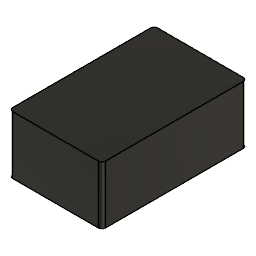
CRTC2025场地（发加工版）V0.1 (Autodesk Fusion 360 archive; units mm, degrees)
design "2*2连接块"
part number: 2025-10-05-20-54-49-775
part number: 2025-10-05-20-58-51-837
part number: 2025-10-05-21-00-41-640
Autodesk Fusion 360 part; units mm, degrees
note: some values were not read from the file. Chosen so that the rebuilt part matches the saved one: which bodies a step acts on.
sketch "草图1" plane through (0, 0, 0) normal (0, 0, 1) x (1, 0, 0)
  line L0 (-16, 25) -> (16, 25)
  line L1 (16, 25) -> (16, -25)
  line L2 (16, -25) -> (-16, -25)
  line L3 (-16, -25) -> (-16, 25)
  line L4 (-16, 25) -> (16, -25) construction
  line L5 (16, 25) -> (-16, -25) construction
  dimension "d1" = 50
  dimension "d2" = 32
  constraint horizontal L0
  constraint perpendicular L0 L1
  constraint parallel L0 L2
  constraint parallel L1 L3
  constraint coincident L4 origin
  constraint coincident L5 origin
  measures "d1" distance of L0.end L1.end
  measures "d2" distance of L1.end L2.end
extrude "拉伸1" add sketch "草图1" along normal blind 20 makes body 1
sketch "草图2" plane through (0, 0, 0) normal (0, 0, -1) x (1, 0, 0)
  line L0 (16, 25) -> (-16, 25)
  line L1 (-16, 25) -> (-16, -25)
  line L2 (-16, -25) -> (16, -25)
  line L3 (16, -25) -> (16, 25)
  line L4 (0, 25) -> (0, -25) construction
  line L5 (0, 0) -> (-16, 0) construction
  circle A0 centre (-8, 12.5) radius 4.05
  circle A1 centre (-8, -12.5) radius 4.05
  circle A2 centre (8, 12.5) radius 4.05
  circle A3 centre (8, -12.5) radius 4.05
  dimension "d5" = 25
  dimension "d6" = 8.1
  dimension "d7" = 16
  constraint midpoint L0 L4.start
  constraint midpoint L2 L4.end
  constraint coincident L5.start origin
  constraint midpoint L1 L5.end
  constraint symmetric L5 A0 A1
  constraint symmetric L4 A0 A2
  constraint symmetric L4 A1 A3
  measures "d5" distance of A0.centre A1.centre
  measures "d6" diameter of A0
  measures "d7" distance of A0.centre A2.centre
extrude "拉伸2" cut sketch "草图2" against normal blind 5.2 contours A0 | A1 | A2 | A3 bodies 1
chamfer "倒角1" distance 0.5 angle 45 4 edges at (-11.7759, -13.9645, 0) (4.2241, -13.9645, 0) (4.2241, 11.0355, 0) (-11.7759, 11.0355, 0) measured on face at (-1.9917, -2.9975, 0) measured on face at (-1.9917, -2.9975, 0) measured on face at (-1.9917, -2.9975, 0) measured on face at (-1.9917, -2.9975, 0) on bodies 1
copy_body "实体->零部件1" bodies 1 removing the originals makes body 2 in component "磁吸连接块"
fillet "圆角1" radius 1.2 4 edges at (-16, -25, 10) (-16, 25, 10) (16, 25, 10) (16, -25, 10) on bodies 2 in component "磁吸连接块"
sketch "草图3" plane through (0, 0, 5.2) normal (0, 0, -1) x (1, 0, 0)
  circle A0 centre (-8, -12.5) radius 4.05
  circle A1 centre (-8, -12.5) radius 4
  dimension "d14" = 8
  constraint concentric A0 A1
  measures "d14" diameter of A1
extrude "拉伸1'" add sketch "草图3" along normal blind 5 from surface at 0.2 separate body contours A1 makes body 3 in component "8*5铷磁铁"
chamfer "倒角1'" distance 0.2 angle 45 2 edges at (-11.7293, 13.9465, 0) (-11.7293, 13.9465, 5) measured on face at (-6.2388, 11.5344, 0) measured on face at (-4.005, 12.6994, 1.6667) on bodies 3 in component "8*5铷磁铁"
pattern_linear "00000000-0000-0000-0000-000000000000" [suppressed]
component "磁吸连接块" placed x (1, 0, 0) y (0, 1, 0) z (0, 0, 1) at (0, 0, 0)
component "8*5铷磁铁" placed x (1, 0, 0) y (0, 1, 0) z (0, 0, 1) at (0, 0, 0)
component "8*5铷磁铁" placed x (1, 0, 0) y (0, 1, 0) z (0, 0, 1) at (16, 0, 0)
component "8*5铷磁铁" placed x (1, 0, 0) y (0, 1, 0) z (0, 0, 1) at (0, -25, 0)
component "8*5铷磁铁" placed x (1, 0, 0) y (0, 1, 0) z (0, 0, 1) at (16, -25, 0)

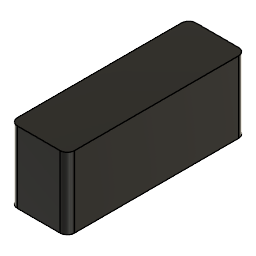
design "2*1连接块"
part number: 2025-10-05-21-16-30-813
part number: 2025-10-05-21-19-39-389
part number: 2025-10-05-21-19-51-506
Autodesk Fusion 360 part; units mm, degrees
sketch "草图1" plane through (0, 0, 0) normal (0, 0, 1) x (1, 0, 0)
  line L0 (-8, 25) -> (8, 25)
  line L1 (8, 25) -> (8, -25)
  line L2 (8, -25) -> (-8, -25)
  line L3 (-8, -25) -> (-8, 25)
  line L4 (-8, 25) -> (8, -25) construction
  line L5 (8, 25) -> (-8, -25) construction
  dimension "d1" = 16
  dimension "d2" = 50
  constraint horizontal L0
  constraint perpendicular L0 L1
  constraint parallel L0 L2
  constraint parallel L1 L3
  constraint coincident L4 origin
  constraint coincident L5 origin
  measures "d1" distance of L1.end L2.end
  measures "d2" distance of L0.end L1.end
extrude "拉伸1" add sketch "草图1" along normal blind 20 makes body 1
sketch "草图2" plane through (0, 0, 0) normal (0, 0, -1) x (1, 0, 0)
  line L0 (8, 25) -> (-8, 25)
  line L1 (-8, 25) -> (-8, -25)
  line L2 (-8, -25) -> (8, -25)
  line L3 (8, -25) -> (8, 25)
  line L4 (0, 25) -> (0, -25) construction
  line L5 (-8, 0) -> (8, 0) construction
  circle A0 centre (0, 12.5) radius 4.05
  circle A1 centre (0, -12.5) radius 4.05
  dimension "d5" = 25
  dimension "d6" = 8.1
  constraint midpoint L0 L4.start
  constraint midpoint L2 L4.end
  constraint midpoint L1 L5.start
  constraint midpoint L3 L5.end
  constraint coincident L4 A0.centre
  constraint symmetric L5 A0 A1
  measures "d5" distance of A0.centre A1.centre
  measures "d6" diameter of A0
extrude "拉伸2" cut sketch "草图2" against normal blind 5.2 contours A0 | A1 bodies 1
fillet "圆角1" radius 2 4 edges at (-8, -25, 10) (-8, 25, 10) (8, 25, 10) (8, -25, 10) on bodies 1
chamfer "倒角1" distance 0.5 angle 45 2 edges at (-3.7759, -13.9645, 0) (-3.7759, 11.0355, 0) measured on face at (0.1009, -22.1796, 0) measured on face at (0.1009, -22.1796, 0) on bodies 1
copy_body "实体->零部件1" bodies 1 removing the originals makes body 2 in component "2*1连接块"
sketch "草图3" plane through (0, 0, 5.2) normal (0, 0, -1) x (1, 0, 0)
  circle A0 centre (0, 12.5) radius 4
  circle A1 centre (0, 12.5) radius 4.05
  circle A2 centre (0, 12.5) radius 4.05
  dimension "d13" = 8
  constraint concentric A0 A1
  measures "d13" diameter of A0
extrude "拉伸1'" add sketch "草图3" along normal blind 5 from surface at 0.2 separate body contours A0 makes body 3 in component "8*5铷磁铁"
chamfer "倒角1'" distance 0.2 angle 45 2 edges at (-3.7293, -11.0535, 5) (-3.7293, -11.0535, 0) measured on face at (3.995, -12.3006, 1.6667) measured on face at (0.7803, -13.4366, 0) on bodies 3 in component "8*5铷磁铁"
pattern_linear "00000000-0000-0000-0000-000000000000" [suppressed]
component "2*1连接块" placed x (1, 0, 0) y (0, 1, 0) z (0, 0, 1) at (0, 0, 0)
component "8*5铷磁铁" placed x (1, 0, 0) y (0, 1, 0) z (0, 0, 1) at (0, 0, 0)
component "8*5铷磁铁" placed x (1, 0, 0) y (0, 1, 0) z (0, 0, 1) at (0, 25, 0)

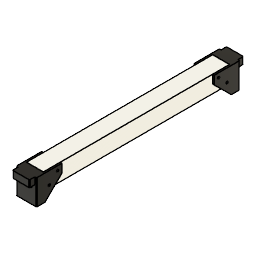
design "桥梁方案1"
part number: 2025-10-07-00-57-18-656
part number: 2025-10-07-01-01-07-836
part number: 2025-10-07-01-23-57-866
part number: 2025-10-07-01-26-28-886
Autodesk Fusion 360 part; units mm, degrees
sketch "草图1" plane through (0, 0, 0) normal (0, 1, 0) x (1, 0, 0)
  line L0 (-25, -25) -> (25, -25)
  line L1 (25, -25) -> (25, 25)
  line L2 (25, 25) -> (-25, 25)
  line L3 (-25, 25) -> (-25, -25)
  line L4 (-25, -25) -> (25, 25) construction
  line L5 (25, -25) -> (-25, 25) construction
  dimension "d1" = 50
  dimension "d2" = 50
  constraint horizontal L0
  constraint perpendicular L0 L1
  constraint parallel L0 L2
  constraint parallel L1 L3
  constraint coincident L4 origin
  constraint coincident L5 origin
  measures "d1" distance of L0.start L2.end
  measures "d2" distance of L0.start L0.end
extrude "拉伸1" add sketch "草图1" along normal mid plane 550 makes body 1
copy_body "实体->零部件1" bodies 1 removing the originals makes body 2 in component "桥体"
sketch "草图2" plane through (0, 275, 0) normal (0, 1, 0) x (-1, 0, 0)
  line L0 (25, -25) -> (25, 25)
  line L1 (25, 25) -> (-25, 25)
  line L2 (-25, 25) -> (-25, -25)
  line L3 (-25, -25) -> (25, -25)
  line L4 (-30, 25) -> (30, 25)
  line L5 (30, 25) -> (30, -30)
  line L6 (30, -30) -> (-30, -30)
  line L7 (-30, -30) -> (-30, 25)
  line L8 (-30, 25) -> (30, -30) construction
  line L9 (30, 25) -> (-30, -30) construction
  point P0 (0, -2.5)
  dimension "d5" = 5
  dimension "d6" = 5
  dimension "d7" = 5
  constraint horizontal L4
  constraint perpendicular L4 L5
  constraint parallel L4 L6
  constraint parallel L5 L7
  constraint coincident L8 P0
  constraint coincident L9 P0
  constraint collinear L1 L4
  measures "d5" distance of L2 L7
  measures "d6" distance of L0 L5
  measures "d7" distance of L3 L6
  measures "d50" diameter of L2.end
  measures "d55" diameter of L2.end
  measures "d62" diameter of L2.end
extrude "拉伸2" add sketch "草图2" against normal blind 50 separate body contours L0 L2 L3 L4 L5 L6 L7 makes body 3
sketch "草图3" plane through (0, 275, 0) normal (0, 1, 0) x (-1, 0, 0)
  line L0 (-30, -30) -> (30, -30)
  line L1 (30, -30) -> (30, 25)
  line L2 (30, 25) -> (25, 25)
  line L3 (25, 25) -> (25, -25)
  line L4 (25, -25) -> (-25, -25)
  line L5 (-25, -25) -> (-25, 25)
  line L6 (-25, 25) -> (-30, 25)
  line L7 (-30, 25) -> (-30, -30)
  line L8 (-30, 25) -> (30, 25)
  line L9 (30, 25) -> (30, -30)
  line L10 (30, -30) -> (-30, -30)
  line L11 (-30, -30) -> (-30, 25)
  constraint horizontal L8
  constraint vertical L9
  constraint horizontal L10
  constraint vertical L11
  constraint coincident L0.end L1.start
  constraint coincident L6.end L7.start
extrude "拉伸3" add sketch "草图3" along normal blind 25 bodies 3
sketch "草图4" plane through (0, 300, 0) normal (0, 1, 0) x (-1, 0, 0)
  line L0 (-30, -30) -> (30, -30)
  line L1 (30, -30) -> (30, 25)
  line L2 (30, 25) -> (-30, 25)
  line L3 (-30, 25) -> (-30, -30)
  line L4 (-30, 25) -> (30, 25)
  line L5 (30, 25) -> (30, 5)
  line L6 (30, 5) -> (-30, 5)
  line L7 (-30, 5) -> (-30, 25)
  dimension "d12" = 20
  constraint horizontal L4
  constraint vertical L5
  constraint horizontal L6
  constraint vertical L7
  constraint coincident L1 L5.end
  constraint coincident L2.end L3.start
  measures "d12" distance of L1.end L5.end
extrude "拉伸4" add sketch "草图4" along normal blind 16 contours L1 L2 L3 L4 L5 L6 L7 bodies 3
sketch "草图6" plane through (30, 0, 0) normal (1, 0, 0) x (0, 1, 0)
  line L0 (316, 25) -> (225, 25)
  line L1 (225, 25) -> (225, -30)
  line L2 (225, -30) -> (300, -30)
  line L3 (300, -30) -> (300, 5)
  line L4 (300, 5) -> (316, 5)
  line L5 (316, 5) -> (316, 25)
  line L6 (316, 5) -> (300, 5)
  line L7 (300, 5) -> (300, 25)
  line L8 (300, 25) -> (316, 25)
  line L9 (316, 25) -> (316, 5)
  constraint horizontal L6
  constraint vertical L7
  constraint horizontal L8
  constraint vertical L9
  constraint coincident L0 L7.end
  constraint coincident L4.end L5.start
  constraint collinear L3 L7
extrude "拉伸5" cut sketch "草图6" against normal blind 5 contours L0 L4 L5 L6 L7 L8 L9 bodies 3
mirror "镜像1" about plane through (0, 0, 0) normal (1, 0, 0) of "拉伸5"
sketch "草图5" plane through (0, 0, 5) normal (0, 0, -1) x (1, 0, 0)
  line L0 (25, -300) -> (-25, -300)
  line L1 (-25, -316) -> (25, -316)
  line L2 (25, -308) -> (-25, -308) construction
  line L3 (0, -316) -> (0, -300) construction
  circle A0 centre (12.5, -308) radius 4.05
  circle A1 centre (-12.5, -308) radius 4.05
  line L4 (-25, -300) -> (-25, -316)
  line L5 (25, -316) -> (25, -300)
  dimension "d20" = 25
  dimension "d21" = 8.1
  constraint midpoint L1 L3.start
  constraint midpoint L0 L3.end
  constraint coincident L2 A0.centre
  constraint coincident L2 A1.centre
  constraint symmetric L3 A0 A1
  constraint midpoint L2.start L5
  constraint perpendicular L2 L5
  constraint midpoint L2.end L4
  measures "d20" distance of A0.centre A1.centre
  measures "d21" diameter of A0
extrude "拉伸6" cut sketch "草图5" against normal blind 5.2 contours A0 | A1 bodies 3
chamfer "倒角1" distance 0.5 angle 45 2 edges at (8.7241, 306.5355, 5) (-16.2759, 306.5355, 5) on bodies 3
sketch "草图7" plane through (30, 0, 0) normal (1, 0, 0) x (0, 1, 0)
  line L0 (300, -30) -> (300, 25)
  line L1 (300, 25) -> (225, 25)
  line L2 (225, 25) -> (225, -30)
  line L3 (225, -30) -> (300, -30)
  line L4 (275, 25) -> (225, 25) construction
  line L5 (225, 25) -> (275, 25) construction
  line L6 (275, 25) -> (275, -25) construction
  line L7 (275, -25) -> (225, -25) construction
  line L8 (225, -25) -> (225, 25) construction
  line L9 (225, 25) -> (275, -25) construction
  line L10 (275, 25) -> (225, -25) construction
  circle A0 centre (237.6256, 12.3744) radius 1.5
  circle A1 centre (262.3744, -12.3744) radius 1.5
  dimension "d27" = 50
  dimension "d28" = 3
  dimension "d29" = 35
  constraint horizontal L5
  constraint vertical L6
  constraint horizontal L7
  constraint vertical L8
  constraint coincident L1.end L2.start
  constraint coincident L4.start L5.end
  constraint coincident L9 A0.centre
  constraint symmetric L10 A0 A1
  measures "d27" distance of L4.start L6.end
  measures "d28" diameter of A0
  measures "d29" distance of A0.centre A1.centre
extrude "拉伸7" cut sketch "草图7" against normal blind 4 contours A0 | A1 bodies 3
sketch "草图8" plane through (30, 0, 0) normal (1, 0, 0) x (0, 1, 0)
  circle A0 centre (237.6256, 12.3744) radius 1.5
  circle A1 centre (262.3744, -12.3744) radius 1.5
  line L0 (300, -30) -> (300, 25)
  line L1 (300, 25) -> (225, 25)
  line L2 (225, 25) -> (225, -30)
  line L3 (225, -30) -> (300, -30)
  line L4 (225, 0) -> (255, -30)
  dimension "d32" = 45
  dimension "d33" = 25
  constraint coincident L2 L4.start
  constraint coincident L3 L4.end
  measures "d32" angle of L2 L4
  measures "d33" distance of L1.end L4.start
extrude "拉伸8" cut sketch "草图8" against normal up to surface (60 mm away) contours L2 L3 L4 bodies 3
sketch "草图9" plane through (30, 0, 0) normal (1, 0, 0) x (0, 1, 0)
  line L0 (225, 0) -> (255, -30)
  line L1 (255, -30) -> (300, -30)
  line L2 (300, -30) -> (300, 25)
  line L3 (300, 25) -> (225, 25)
  line L4 (225, 25) -> (225, 0)
  circle A0 centre (262.3744, -12.3744) radius 1.5
  circle A1 centre (237.6256, 12.3744) radius 1.5
  line L5 (255, -30) -> (275, -50)
  line L6 (275, -50) -> (300, -50)
  line L7 (300, -50) -> (300, -30)
  dimension "d36" = 20
  constraint coincident L0.end L1.start
  constraint parallel L0 L5
  constraint parallel L1 L6
  constraint coincident L1.end L2.start
  constraint perpendicular L1 L7
  measures "d36" distance of L1 L6
extrude "拉伸9" add sketch "草图9" against normal blind 60 contours L1 L5 L6 L7 bodies 3
sketch "草图10" plane through (0, 0, -50) normal (0, 0, -1) x (1, 0, 0)
  line L0 (30, -300) -> (30, -275)
  line L1 (30, -275) -> (-30, -275)
  line L2 (-30, -275) -> (-30, -300)
  line L3 (-30, -300) -> (30, -300)
  line L4 (0, -300) -> (0, -275) construction
  line L5 (25, -294) -> (-25, -294)
  line L6 (-25, -294) -> (-25, -254)
  line L7 (-25, -254) -> (25, -254)
  line L8 (25, -254) -> (25, -294)
  line L9 (25, -294) -> (-25, -254) construction
  line L10 (-25, -294) -> (25, -254) construction
  point P0 (0, -274)
  dimension "d39" = 6
  dimension "d40" = 5
  dimension "d41" = 40
  constraint midpoint L3 L4.start
  constraint midpoint L1 L4.end
  constraint horizontal L5
  constraint perpendicular L5 L6
  constraint parallel L5 L7
  constraint parallel L6 L8
  constraint coincident L9 P0
  constraint coincident L10 P0
  constraint coincident L4 P0
  measures "d39" distance of L3 L5
  measures "d40" distance of L0 L8
  measures "d41" distance of L5 L7
extrude "拉伸10" cut sketch "草图10" against normal blind 20 contours L1 L5 L6 L8 | L1 L6 L7 L8 bodies 3
fillet "圆角2" radius 3 6 edges at (25, 294, -40) (-25, 294, -40) (27.5, 225, 0) (-27.5, 225, 0) (-27.5, 275, -50) (27.5, 275, -50) on bodies 3
mirror "镜像2" about plane through (0, 0, 0) normal (1, 0, 0) of "拉伸7"
sketch "草图11" plane through (0, 300, 0) normal (0, 1, 0) x (-1, 0, 0)
  line L0 (25, 5) -> (-25, 5)
  line L1 (-25, 5) -> (-25, 25)
  line L2 (-25, 25) -> (-30, 25)
  line L3 (-30, 25) -> (-30, -50)
  line L4 (-30, -50) -> (30, -50)
  line L5 (30, -50) -> (30, 25)
  line L6 (30, 25) -> (25, 25)
  line L7 (25, 25) -> (25, 5)
  line L8 (-30, -5) -> (30, -5) construction
  circle A0 centre (-12.5, -5) radius 3.1
  line L9 (0, 0) -> (0, -5) construction
  circle A1 centre (12.5, -5) radius 3.1
  dimension "d49" = 5
  dimension "d50" = 6.2
  dimension "d51" = 25
  constraint coincident L3 L8.start
  constraint coincident L5 L8.end
  constraint perpendicular L5 L8
  constraint coincident L8 A0.centre
  constraint coincident L9.start origin
  constraint midpoint L8 L9.end
  constraint symmetric A0 L9 A1
  measures "d49" distance of L9.start L8
  measures "d50" diameter of A0
  measures "d51" distance of A0.centre A1.centre
extrude "拉伸11" cut sketch "草图11" against normal blind 5 contours A0 | A1 bodies 3
chamfer "倒角2" distance 0.5 angle 45 2 edges at (15.3902, 300, -3.879) (-9.6098, 300, -3.879) on bodies 3
sketch "草图12" plane through (0, 295, 0) normal (0, 1, 0) x (-1, 0, 0)
  circle A0 centre (-12.5, -5) radius 3.1
  circle A1 centre (-12.5, -5) radius 1.6
  dimension "d55" = 3.2
  constraint concentric A0 A1
  measures "d55" diameter of A1
extrude "拉伸12" cut sketch "草图12" against normal through all contours A1 bodies 3
mirror "镜像3" about plane through (0, 0, 0) normal (1, 0, 0) of "拉伸12"
fillet "圆角3" radius 2 4 edges at (25, 316, 15) (-25, 316, 15) (30, 300, -12.5) (-30, 300, -12.5) on bodies 3
chamfer "倒角3" distance 1.8 angle 45 4 edges at (30, 236.2271, 12.9168) (30, 260.9759, -11.8319) (-30, 236.2271, 11.8319) (-30, 260.9759, -12.9168) on bodies 3
copy_body "实体->零部件2" bodies 3 removing the originals makes body 4 in component "桥梁磁吸件"
mirror "镜像零部件1" about plane through (0, 0, 0) normal (0, 0, 1) of bodies 4 makes body 5 in component "桥梁磁吸件(镜像)"
sketch "草图13" plane through (0, 0, 10.2) normal (0, 0, -1) x (1, 0, 0)
  circle A0 centre (-12.5, 308) radius 4.05
  circle A1 centre (-12.5, 308) radius 4
  dimension "d62" = 8
  constraint concentric A0 A1
  measures "d62" diameter of A1
extrude "拉伸1'" add sketch "草图13" along normal blind 5 from surface at 0.2 separate body contours A1 makes body 6 in component "8*5铷磁铁"
chamfer "倒角1'" distance 0.2 angle 45 2 edges at (-16.2293, -306.5535, 10) (-16.2293, -306.5535, 5) on bodies 6 in component "8*5铷磁铁"
pattern_linear "R-阵列1" count 2 spacing 25 along (1, 0, 0) count 2 spacing 616 along (0, 1, 0) of bodies 6 makes body 7 at (8.5793, -308.7926, 6.7333) makes body 8 at (-16.4207, 307.2074, 6.7333) makes body 9 at (8.5793, 307.2074, 6.7333) in component "8*5铷磁铁"
component "桥体" placed x (1, 0, 0) y (0, 1, 0) z (0, 0, 1) at (0, 0, 0)
component "桥梁磁吸件" placed x (1, 0, 0) y (0, 1, 0) z (0, 0, 1) at (0, 0, 0)
component "桥梁磁吸件(镜像)" placed x (1, 0, 0) y (0, -1, 0) z (0, 0, -1) at (0, 0, 0)
component "8*5铷磁铁" placed x (1, 0, 0) y (0, 1, 0) z (0, 0, 1) at (0, 0, 0)
named bodies: "桥体", "桥梁磁吸件"
